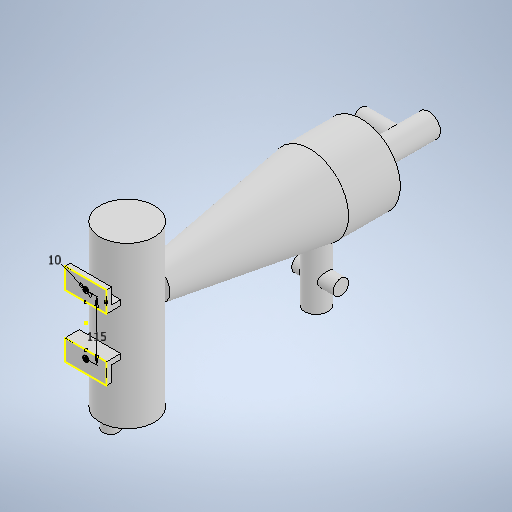
# Autodesk Inventor part: Гидроциклон
Saved by Autodesk Inventor 2025.3 (Build 293356030, 356C)
## iProperties
Created: 2025-08-30
Part Number: Гидроциклон
Material: Generic
Document SubType Name: Modeling
Designer: admin
Density: 1 g/cm^3
Appearance: Default
Author: admin
Autodesk Inventor part; units mm, degrees
ref_plane "YZ Plane" through (0, 0, 0) normal (1, 0, 0) x (0, 1, 0)
ref_plane "XZ Plane" through (0, 0, 0) normal (0, 1, 0) x (-1, 0, 0)
ref_plane "XY Plane" through (0, 0, 0) normal (0, 0, 1) x (1, 0, 0)
sketch "Sketch1" plane through (0, 0, 0) normal (0, 0, 1) x (1, 0, 0)
  circle A0 centre (0, 80) radius 52.5
  point P0 (0, 0)
  dimension "d0" = 105
  dimension "d5" = 80
  constraints: 1 centre point, 1 vertical alignment
  measures "d0" diameter of A0
  measures "d5" distance of point (0, 0) A0.centre
extrude "Extrusion1" add sketch "Sketch1" along normal blind 130 and the other way blind 180
sketch "Sketch2" plane through (0, 0, 0) normal (1, 0, 0) x (0, 1, 0)
  line L0 (132.5, -180) -> (132.5, 130) projected
  line L1 (132.5, 0) -> (662.5, 0)
  line L2 (662.5, 0) -> (662.5, -22.5)
  line L3 (662.5, -22.5) -> (532.5, -22.5)
  line L4 (532.5, -22.5) -> (532.5, -75)
  line L5 (532.5, -75) -> (432.5, -75)
  line L6 (432.5, -75) -> (132.5, -30)
  point P0 (0, 0)
  point P1 (397.5, 0)
  dimension "d6" = 530
  dimension "d8" = 45
  dimension "d9" = 130
  dimension "d10" = 150
  dimension "d11" = 30
  dimension "d12" = 100
  constraints: 12 end point, 3 perpendicular, 2 point on line, 1 horizontal, 1 horizontal alignment, 1 midpoint, 1 vertical
  measures "d6" distance of L1.start L1.end
  measures "d8" diameter of L3 L1
  measures "d9" distance of L2.end L3.end
  measures "d10" diameter of L5 L1
  measures "d11" distance of L1.start L6.end
  measures "d12" distance of L4.end L5.end
revolve "Revolution1" add sketch "Sketch2" angle 360 about axis through (0, 132.5, 0) along (0, 1, 0)
sketch "Sketch3" plane through (0, 0, 0) normal (1, 0, 0) x (0, 1, 0)
  line L0 (27.5, -180) -> (27.5, 130) projected
  line L1 (27.5, 35) -> (0, 35)
  line L2 (0, 35) -> (0, 75)
  line L3 (0, 75) -> (10, 75)
  line L4 (10, 75) -> (10, 45)
  line L5 (10, 45) -> (27.5, 45)
  line L6 (27.5, -45) -> (0, -45)
  line L7 (0, -45) -> (0, -85)
  line L8 (0, -85) -> (10, -85)
  line L9 (10, -85) -> (10, -55)
  line L10 (10, -55) -> (27.5, -55)
  line L11 (132.5, 130) -> (27.5, 130) projected
  point P0 (0, 0)
  point P1 (0, 55)
  point P2 (13.75, 35)
  dimension "d14" = 95
  dimension "d15" = 10
  dimension "d16" = 10
  dimension "d17" = 10
  dimension "d18" = 80
  dimension "d19" = 40
  dimension "d20" = 160
  constraints: 20 end point, 10 perpendicular, 4 point on line, 3 collinear, 2 midpoint, 1 vertical alignment
  measures "d14" distance between parallel lines of L1 L11
  measures "d15" distance between parallel lines of L1 L5
  measures "d16" distance between parallel lines of L6 L10
  measures "d17" distance between parallel lines of L2 L4
  measures "d18" distance from line of L6 point (13.75, 35)
  measures "d19" distance of L1.end L2.end
  measures "d20" distance between parallel lines of L3 L8
extrude "Extrusion2" add sketch "Sketch3" along normal mid plane 80
sketch "Sketch4" plane through (-40, 0, 35) normal (0, -1, 0) x (1, 0, 0)
  line L0 (0, 0) -> (80, 0) projected
  line L1 (80, 40) -> (80, 0) projected
  line L2 (0, 40) -> (80, 40) projected
  line L3 (0, 0) -> (0, 40) projected
  line L4 (0, -120) -> (80, -120) projected
  line L5 (80, -80) -> (80, -120) projected
  line L6 (0, -80) -> (80, -80) projected
  line L7 (0, -120) -> (0, -80) projected
  circle A0 centre (40, -95) radius 5
  circle A1 centre (40, 20) radius 5
  point P0 (40, -35)
  point P1 (80, 20)
  point P2 (40, 0)
  point P3 (40, -80)
  dimension "d23" = 115
  dimension "d24" = 10
  constraints: 3 midpoint, 2 centre point, 2 vertical alignment, 1 equal radius, 1 horizontal alignment
  measures "d23" distance of A0.centre A1.centre
  measures "d24" diameter of A1
sketch "Sketch5" plane through (0, 0, 0) normal (0, 0, 1) x (1, 0, 0)
  line L0 (75, 532.5) -> (-75, 532.5) projected
  line L1 (75, 432.5) -> (-75, 432.5) projected
  circle A0 centre (-47.1676, 492.5) radius 22.5
  point P0 (0, 0)
  point P1 (0, 532.5)
  dimension "d25" = 45
  dimension "d26" = 47.1676
  dimension "d27" = 40
  constraints: 1 centre point, 1 midpoint
  measures "d25" diameter of A0
  measures "d26" horizontal distance of point (0, 532.5) A0.centre
  measures "d27" distance from line of L0 A0.centre
extrude "Extrusion3" add sketch "Sketch5" against normal blind 240
sketch "Sketch6" plane through (0, 80, -180) normal (0, 0, -1) x (-1, 0, 0)
  circle A0 centre (0, -31.9498) radius 15
  point P0 (0, -80)
  dimension "d30" = 30
  constraints: 1 centre point
  measures "d30" diameter of A0
extrude "Extrusion4" add sketch "Sketch6" along normal blind 20
sketch "Sketch7" plane through (0, 0, 0) normal (1, 0, 0) x (0, 1, 0)
  line L0 (662.5, -22.5) -> (662.5, 22.5) projected
  line L1 (532.5, -22.5) -> (532.5, 22.5) projected
  line L2 (470, -240) -> (515, -240) projected
  circle A0 centre (612.2809, 0) radius 15
  circle A1 centre (492.5, -186.3379) radius 15
  point P0 (0, 0)
  dimension "d33" = 30
  dimension "d34" = 30
  constraints: 2 centre point, 1 other
  measures "d33" diameter of A1
  measures "d34" diameter of A0
extrude "Extrusion5" add sketch "Sketch7" against normal blind 80
equation "\"d16\" = d15"
equation "\"d17\" = d15"
body "Solid1"
